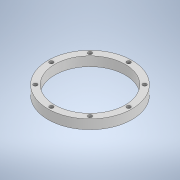
# Autodesk Inventor part: Adapter_bearing_joint
Saved by Autodesk Inventor 2021 (Build 250183000, 183)
## iProperties
Created: 2020-05-19
Part Number: Adapter_bearing_joint
Material: Generic
Document SubType Name: Modeling
Designer: Motius
Density: 1 g/cm^3
Appearance: Default
Author: Motius
Autodesk Inventor part; units mm, degrees
ref_plane "YZ Plane" through (0, 0, 0) normal (1, 0, 0) x (0, 1, 0)
ref_plane "XZ Plane" through (0, 0, 0) normal (0, 1, 0) x (-1, 0, 0)
ref_plane "XY Plane" through (0, 0, 0) normal (0, 0, 1) x (1, 0, 0)
sketch "Sketch1" plane through (0, 0, 0) normal (0, 0, 1) x (1, 0, 0)
  line L0 (0, 7.7) -> (0, -7.7) construction
  line L1 (-9.9, 0) -> (59.4, 0) construction
  line L2 (41.5, 5.5) -> (41.5, -5.5)
  line L3 (41.5, -5.5) -> (49.5, -5.5)
  line L4 (49.5, -5.5) -> (49.5, 5.5)
  line L5 (49.5, 5.5) -> (41.5, 5.5)
  line L6 (45.5, 5.5) -> (45.5, -5.5) construction
  point P0 (0, 0)
  dimension "d0" = 45.5
  dimension "d1" = 4
  dimension "d2" = 11
  constraints: 10 end point, 3 perpendicular, 2 midpoint, 1 vertical, 1 other
  measures "d0" distance between parallel lines of L0 L6
  measures "d1" distance between parallel lines of L2 L6
  measures "d2" distance between parallel lines of L3 L5
revolve "Revolution1" add sketch "Sketch1" angle 360 about axis through (0, 0, 0) along (0, -1, 0)
sketch "Sketch2" plane through (0, 5.5, 0) normal (0, 1, 0) x (1, 0, 0)
  line L0 (0, 69.3) -> (0, -69.3) construction
  line L1 (69.3, 0) -> (-69.3, 0) construction
  circle A0 centre (0, 0) radius 45.5 construction
  circle A1 centre (0, 0) radius 49.5 construction
  circle A2 centre (0, 0) radius 41.5 construction
  point P0 (-45.5, 0)
  point P1 (-32.1734, -32.1734)
  point P2 (0, -45.5)
  point P3 (32.1734, -32.1734)
  point P4 (45.5, 0)
  point P5 (32.1734, 32.1734)
  point P6 (0, 45.5)
  point P7 (-32.1734, 32.1734)
  dimension "d4" = 4
  dimension "d5" = 4
  dimension "d8" = 360
  constraints: 1 coincident, 1 horizontal alignment, 1 point on line, 11 other
hole "Hole1" at (-45.5, 5.5, 0) at (-32.1734, 5.5, 32.1734) at (0, 5.5, 45.5) at (32.1734, 5.5, 32.1734) at (45.5, 5.5, 0) at (32.1734, 5.5, -32.1734) at (0, 5.5, -45.5) at (-32.1734, 5.5, -32.1734) direction (0, -1, 0) diameter 4.5 depth 11.8 tip angle 118 clearance for "Flat Head Machine Screw" size "M4" standard "Ansi Metric M Profile"
equation "\"d4\" = d5"
body "Solid1"
